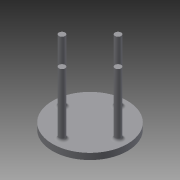
# Autodesk Inventor part: soporte-botella
Saved by Autodesk Inventor 2015 SP1 (Build 190203100, 203)
## iProperties
Created: 2015-06-29
Part Number: soporte-botella
Material: Genérico
Document SubType Name: Modeling
Designer: Javier
Density: 1 g/cm^3
Appearance: Valor por defecto
Author: Javier
Autodesk Inventor part; units mm, degrees
ref_plane "YZ Plane" through (0, 0, 0) normal (1, 0, 0) x (0, 1, 0)
ref_plane "XZ Plane" through (0, 0, 0) normal (0, 1, 0) x (-1, 0, 0)
ref_plane "XY Plane" through (0, 0, 0) normal (0, 0, 1) x (1, 0, 0)
sketch "Boceto1" plane through (0, 0, 0) normal (0, 0, 1) x (1, 0, 0)
  circle A0 centre (0, 0) radius 30
  dimension "d0" = 60
  constraints: 1 centre point, 1 coincident
  measures "d0" diameter of A0
extrude "Extrusión1" add sketch "Boceto1" along normal blind 5
sketch "Boceto2" plane through (0, 0, 5) normal (0, 0, 1) x (1, 0, 0)
  circle A0 centre (0, 0) radius 20
  circle A1 centre (0, 0) radius 25
  line L0 (0, 20) -> (0, 25)
  circle A2 centre (0, 22.5) radius 2.5
  line L1 (20, 0) -> (25, 0)
  circle A3 centre (22.5, 0) radius 2.5
  line L2 (0, -20) -> (0, -25)
  circle A4 centre (0, -22.5) radius 2.5
  line L3 (-25, 0) -> (-20, 0)
  circle A5 centre (-22.5, 0) radius 2.5
  dimension "d3" = 40
  dimension "d4" = 50
  constraints: 8 end point, 8 point on circle, 4 midpoint, 2 centre point, 2 coincident, 2 horizontal, 2 horizontal alignment, 2 vertical, 2 vertical alignment, 8 other
  measures "d3" diameter of A0
  measures "d4" diameter of A1
extrude "Extrusión2" add sketch "Boceto2" along normal blind 50 contours A3 L1 | L1 A3 | A2 L0 | L0 A2 | A4 L2 | L2 A4 | A5 L3 | L3 A5
fillet "Empalme1" radius 2 4 edges at (-2.5, 22.5, 5) (20, 0, 5) (-2.5, -22.5, 5) (-25, 0, 5)
